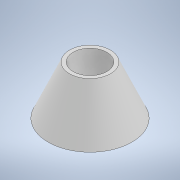
# Autodesk Inventor part: Basis (WIP)
Saved by Autodesk Inventor 2022 (Build 260153000, 153)
## iProperties
Created: 2022-04-26
Part Number: Basis (WIP)
Material: Generic
Document SubType Name: Modeling
Designer: kajve
Density: 1 g/cm^3
Appearance: Default
Author: kajve
Autodesk Inventor part; units mm, degrees
ref_plane "YZ Plane" through (0, 0, 0) normal (1, 0, 0) x (0, 1, 0)
ref_plane "XZ Plane" through (0, 0, 0) normal (0, 1, 0) x (-1, 0, 0)
ref_plane "XY Plane" through (0, 0, 0) normal (0, 0, 1) x (1, 0, 0)
sketch "Sketch1" plane through (0, 0, 0) normal (0, 0, 1) x (1, 0, 0)
  line L0 (0, 0) -> (6.3484, 0)
  line L1 (6.3484, 0) -> (0, 14.5006)
  line L2 (0, 14.5006) -> (0, 0)
  constraints: 6 end point, 1 horizontal, 1 perpendicular
revolve "Revolution1" add sketch "Sketch1" angle 360 about axis through (0, 14.5006, 0) along (0, -1, 0)
ref_plane "Work Plane1" through (30.5852, -3, 9.073) normal (1, 0, 0) x (0, 0, -1)
sketch "Sketch5" plane through (30.5852, -3, 9.073) normal (1, 0, 0) x (0, 0, -1)
  line L0 (0, 23) -> (0, 0) projected
  line L1 (18.1461, 0) -> (0, 0) projected
  line L2 (18.1461, 0) -> (18.1461, 23) projected
  line L3 (0, 23) -> (18.1461, 23) projected
  line L4 (0, 10.3899) -> (18.1461, 10.3899)
  line L5 (18.1461, 10.3899) -> (18.1461, 23)
  line L6 (18.1461, 23) -> (0, 23)
  line L7 (0, 23) -> (0, 10.3899)
  point P0 (9.073, 3)
  constraints: 8 end point, 2 parallel, 1 horizontal, 1 perpendicular, 1 point on line
extrude "Extrusion3" cut sketch "Sketch5" against normal through all contours L3 L2 L4 L0
sketch "Sketch6" plane through (0, 7.3899, 0) normal (0, 1, 0) x (1, 0, 0)
  circle A0 centre (0, 0) radius 3.1131 projected
  circle A1 centre (0, 0) radius 2.5554
  constraints: 1 centre point, 1 coincident
extrude "Extrusion4" cut sketch "Sketch6" against normal through all contours A1
sketch "Sketch7" plane through (0, 0, 0) normal (0, -1, 0) x (1, 0, 0)
  circle A0 centre (0, 0) radius 2.5554 projected
  circle A1 centre (0, 0) radius 6.3484 projected
  circle A2 centre (0, 0) radius 4.0227
  constraints: 1 centre point, 1 coincident
extrude "Extrusion5" cut sketch "Sketch7" against normal blind 3.7 contours A2
sketch "Sketch8" plane through (0, 3.7, 0) normal (0, -1, 0) x (1, 0, 0)
  circle A0 centre (0, 0) radius 4.0227 projected
  circle A1 centre (0, 0) radius 2.5554 projected
sketch "Sketch9" plane through (0, 0, 0) normal (0, -1, 0) x (1, 0, 0)
  circle A0 centre (0, 0) radius 4.0227 projected
  circle A1 centre (0, 0) radius 6.3484 projected
  circle A2 centre (0, 0) radius 5.406
  constraints: 1 centre point, 1 coincident
extrude "Extrusion6" cut sketch "Sketch9" against normal blind 1 contours A2
body "Solid1"
